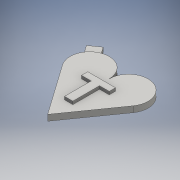
# Autodesk Inventor part: Gift - T
Saved by Autodesk Inventor 2016 (Build 200138000, 138)
## iProperties
Created: 2016-02-04
Part Number: Gift - T
Material: Generic
Document SubType Name: Modeling
Designer: TimB
Density: 1 g/cm^3
Appearance: Default
Author: TimB
Autodesk Inventor part; units mm, degrees
ref_plane "YZ Plane" through (0, 0, 0) normal (1, 0, 0) x (0, 1, 0)
ref_plane "XZ Plane" through (0, 0, 0) normal (0, 1, 0) x (-1, 0, 0)
ref_plane "XY Plane" through (0, 0, 0) normal (0, 0, 1) x (1, 0, 0)
sketch "Sketch1" plane through (0, 0, 0) normal (0, 0, 1) x (1, 0, 0)
  line L0 (0, -14) -> (-11.8124, 2.7546)
  line L1 (0, -14) -> (11.8124, 2.7546)
  arc A0 (0, 6.5) -> (-11.8124, 2.7546) centre (-6.5, 6.5) ccw
  arc A1 (11.8124, 2.7546) -> (0, 6.5) centre (6.5, 6.5) ccw
  point P0 (0, 0)
  constraints: 4 end point, 4 point on circle, 3 tangent, 2 centre point
extrude "Extrusion1" add sketch "Sketch1" along normal blind 2
sketch "Sketch6" plane through (0, 0, 0) normal (0, 0, -1) x (-1, 0, 0)
  line L0 (-11.8124, 2.7546) -> (0, -14) projected
  line L1 (11.8124, 2.7546) -> (0, -14) projected
  line L2 (0, -14) -> (0, -7)
  line L3 (-4.9352, -7) -> (4.9352, -7)
  line L4 (-1.3817, -7) -> (-1.3817, 1.9052)
  line L5 (-1.3817, 1.9052) -> (-4.6353, 1.9052)
  line L6 (-4.6353, 1.9052) -> (-4.6353, 4)
  line L7 (-4.6353, 4) -> (4.6353, 4)
  line L8 (4.6353, 4) -> (4.6353, 1.9052)
  line L9 (4.6353, 1.9052) -> (1.3817, 1.9052)
  line L10 (1.3817, 1.9052) -> (1.3817, -7)
  line L11 (1.3817, -7) -> (-1.3817, -7)
  point P0 (0, 0)
  dimension "d24" = 7
  constraints: 4 end point, 2 horizontal, 2 point on line, 1 vertical
  measures "d24" distance of L0.end L2.end
extrude "Extrusion5" add sketch "Sketch6" against normal blind 3 contours L4 L5 L6 L7 L8 L9 L10 L3
sketch "Sketch7" plane through (0, 0, 0) normal (0, 0, -1) x (-1, 0, 0)
  arc A0 (11.8124, 2.7546) -> (0, 6.5) centre (6.5, 6.5) ccw
  line L0 (10.6694, 15.1841) -> (8.8261, 12.5695)
  line L1 (13.9386, 12.8792) -> (10.6694, 15.1841)
  line L2 (11.9445, 10.0507) -> (13.9386, 12.8792)
  point P0 (0, 0)
  constraints: 6 end point, 2 point on circle, 1 centre point
extrude "Extrusion6" add sketch "Sketch7" against normal blind 1.5
body "Solid1"
